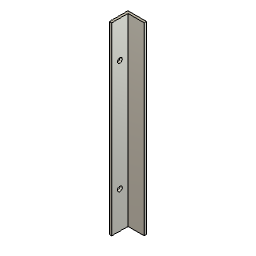
Angle 252 mm Battery Holder v2 (Autodesk Fusion 360 design; units mm, degrees)
Autodesk Fusion 360 part; units mm, degrees
sketch "Sketch1" plane through (0, 0, 0) normal (0, 1, 0) x (1, 0, 0)
  line L0 (0, -25.4) -> (0, 0)
  line L1 (0, 0) -> (25.4, 0)
  line L2 (12.7, -12.7) -> (11.05, -11.05) construction
  line L3 (3.175, -25.4) -> (3.175, -3.175)
  line L4 (3.175, -3.175) -> (25.4, -3.175)
  line L5 (25.4, -3.175) -> (25.4, 0)
  line L6 (0, -25.4) -> (3.175, -25.4)
  dimension "d1" = 25.4
  dimension "d2" = 25.4
  dimension "d13" = 3.175
  constraint coincident L0.end L2
  constraint coincident L0.end L1.start
  constraint perpendicular L1 L5
  constraint vertical L0
  constraint horizontal L1
  measures "d1" distance of L0.end L1.end
  measures "d2" distance of L0.start L0.end
extrude "Extrude1" add sketch "Sketch1" along normal blind 126
hole "Hole3" at (3.175, 76, 14.2875) direction (-1, 0, 0) diameter 6.5 end through all
mirror "Mirror1" about plane through (0, 0, 0) normal (0, 1, 0) of bodies 1 merged
equation "d5 = ( 252 / 2 ) * 1 mm"
equation "d27 = ( 22.225 / 2 ) * 1 mm"
